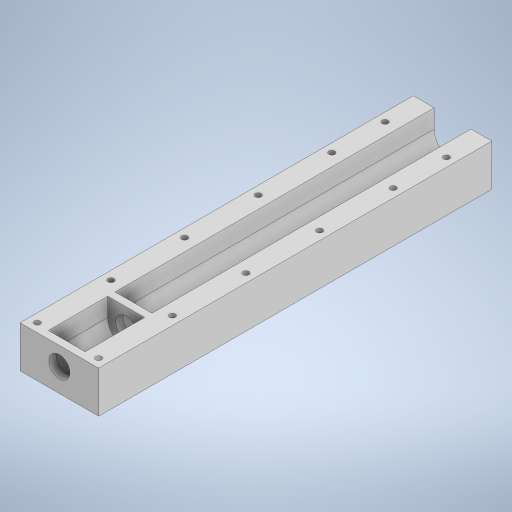
# Autodesk Inventor part: body_v2
Saved by Autodesk Inventor 2023 (Build 270158000, 158)
## iProperties
Created: 2023-07-18
Part Number: body_v2
Material: Generic
Document SubType Name: Modeling
Designer: checo
Density: 1 g/cm^3
Appearance: Default
Author: checo
Autodesk Inventor part; units mm, degrees
ref_plane "YZ Plane" through (0, 0, 0) normal (1, 0, 0) x (0, 1, 0)
ref_plane "XZ Plane" through (0, 0, 0) normal (0, 1, 0) x (-1, 0, 0)
ref_plane "XY Plane" through (0, 0, 0) normal (0, 0, 1) x (1, 0, 0)
sketch "Sketch1" plane through (0, 0, 0) normal (0, 0, 1) x (1, 0, 0)
  circle A0 centre (0, 0) radius 7.5
  line L0 (-16, 7.5) -> (16, 7.5)
  line L1 (16, 7.5) -> (16, -9.5)
  line L2 (16, -9.5) -> (-16, -9.5)
  line L3 (-16, -9.5) -> (-16, 7.5)
  line L4 (-7.5, 0) -> (-7.5, 7.5)
  line L5 (7.5, 0) -> (7.5, 7.5)
  point P0 (0, -9.5)
  dimension "d0" = 15
  dimension "d5" = 32
  dimension "d6" = 2
  constraints: 13 end point, 3 perpendicular, 3 tangent, 2 point on circle, 2 point on line, 1 centre point, 1 coincident, 1 horizontal, 1 midpoint, 1 parallel, 1 vertical, 1 vertical alignment
  measures "d0" diameter of A0
  measures "d5" distance of L1.end L2.end
  measures "d6" distance edge to line of A0 L2
extrude "Extrusion1" add sketch "Sketch1" along normal blind 24.2 contours A0 L5 L0 L1 L2 L3 L4
sketch "Sketch2" plane through (0, 0, 24.2) normal (0, 0, 1) x (1, 0, 0)
  line L0 (-16, -9.5) -> (16, -9.5) projected
  line L1 (16, -9.5) -> (16, 7.5) projected
  line L2 (16, 7.5) -> (7.5, 7.5) projected
  line L3 (7.5, 7.5) -> (7.5, 0) projected
  arc A0 (-7.5, 0) -> (7.5, 0) centre (0, 0) ccw projected
  line L4 (-7.5, 0) -> (-7.5, 7.5) projected
  line L5 (-7.5, 7.5) -> (-16, 7.5) projected
  line L6 (-16, 7.5) -> (-16, -9.5) projected
  circle A1 centre (0, 0) radius 4.25
  line L7 (-7.5, 7.5) -> (-16, 7.5) projected
  line L8 (-7.5, 7.5) -> (7.5, 7.5)
  dimension "d10" = 8.5
  constraints: 2 end point, 1 centre point, 1 coincident, 1 collinear
  measures "d10" diameter of A1
extrude "Extrusion3" add sketch "Sketch2" along normal blind 3
sketch "Sketch4" plane through (0, 0, 0) normal (0, 0, -1) x (-1, 0, 0)
  line L0 (-16, 7.5) -> (-7.5, 7.5) projected
  line L1 (-16, -9.5) -> (-16, 7.5) projected
  line L2 (16, -9.5) -> (-16, -9.5) projected
  line L3 (16, 7.5) -> (16, -9.5) projected
  line L4 (7.5, 7.5) -> (16, 7.5) projected
  line L5 (-7.5, 7.5) -> (7.5, 7.5) projected
  circle A0 centre (0, 0) radius 4.25 projected
extrude "Extrusion4" add sketch "Sketch4" along normal blind 3
sketch "Sketch5" plane through (0, 0, -3) normal (0, 0, -1) x (-1, 0, 0)
  line L0 (16, 7.5) -> (-16, 7.5) projected
  line L1 (16, -9.5) -> (16, 7.5) projected
  line L2 (-16, -9.5) -> (16, -9.5) projected
  line L3 (-16, 7.5) -> (-16, -9.5) projected
  circle A0 centre (0, 0) radius 7.5
  arc A1 (-7.5, 0) -> (7.5, 0) centre (0, 0) ccw projected
  line L4 (7.5, 0) -> (7.5, 7.5)
  line L5 (-16, 7.5) -> (16, 7.5) projected
  line L6 (-7.5, 7.5) -> (-7.5, 0) projected
  line L7 (-7.5, 0) -> (-7.5, 7.5)
  constraints: 4 end point, 3 tangent, 1 centre point, 1 coincident, 1 collinear, 1 perpendicular, 1 point on line
extrude "Extrusion5" add sketch "Sketch5" along normal blind 130 contours L1 L2 L3 L0 L6 A0 L4
sketch "Sketch6" plane through (0, 0, -133) normal (0, 0, -1) x (-1, 0, 0)
  line L0 (0, 0) -> (0, -9.5) construction
  line L1 (16, -9.5) -> (-16, -9.5) construction
  line L2 (-16, 7.5) -> (-16, -9.5) construction
  point P0 (-12.5, -6)
  point P1 (12.5, -6)
  dimension "d17" = 3.5
  dimension "d18" = 3.5
  constraints: 2 end point, 1 midpoint, 1 symmetric about line
  measures "d17" distance from line of point (-12.5, -6) L2
  measures "d18" distance from line of L1 point (-12.5, -6)
hole "Hole1" at (12.5, -6, -133) at (-12.5, -6, -133) direction (0, 0, 1) diameter 2.3813 depth 10 tip angle 118
sketch "Sketch7" plane through (-16, 7.5, 27.2) normal (0, 1, 0) x (1, 0, 0)
  line L0 (16, 0) -> (16, 160.2) construction
  line L1 (32, 160.2) -> (0, 160.2) projected
  line L2 (0, 160.2) -> (0, 0) projected
  line L3 (32, 0) -> (0, 0) projected
  point P0 (16, 27.2)
  point P1 (3.5, 3.5)
  point P2 (3.5, 33.5)
  point P3 (3.5, 63.5)
  point P4 (3.5, 93.5)
  point P5 (3.5, 123.5)
  point P6 (3.5, 145.2)
  point P7 (28.5, 3.5)
  point P8 (28.5, 33.5)
  point P9 (28.5, 63.5)
  point P10 (28.5, 93.5)
  point P11 (28.5, 123.5)
  point P12 (28.5, 145.2)
  dimension "d27" = 3.5
  dimension "d44" = 30
  dimension "d49" = 3.5
  dimension "d50" = 15
  constraints: 6 symmetric about line, 2 end point, 2 midpoint, 1 vertical, 1 vertical alignment, 4 other
  measures "d27" distance from line of L2 point (3.5, 3.5)
  measures "d44" distance of point (3.5, 3.5) point (3.5, 33.5)
  measures "d49" distance from line of L3 point (3.5, 3.5)
  measures "d50" distance from line of L1 point (3.5, 145.2)
hole "Hole3" at (-12.5, 7.5, 23.7) at (-12.5, 7.5, -6.3) at (-12.5, 7.5, -36.3) at (-12.5, 7.5, -66.3) at (-12.5, 7.5, -96.3) at (-12.5, 7.5, -118) at (12.5, 7.5, 23.7) at (12.5, 7.5, -6.3) at (12.5, 7.5, -36.3) at (12.5, 7.5, -66.3) at (12.5, 7.5, -96.3) at (12.5, 7.5, -118) direction (0, -1, 0) diameter 2.3813 depth 10 tip angle 118
body "Solid1"
